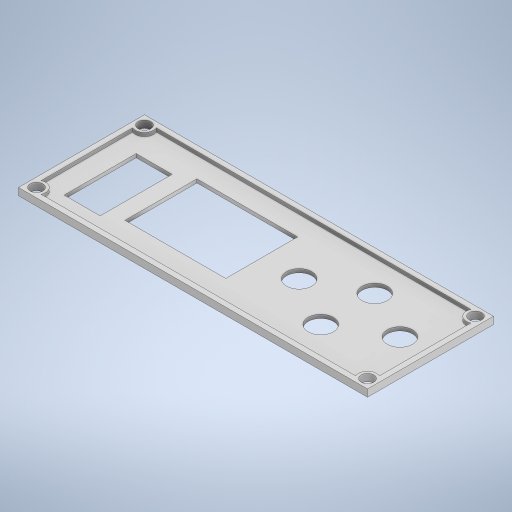
# Autodesk Inventor part: tampa_lcd_botoes
Saved by Autodesk Inventor 2024.3 (Build 283343000, 343)
## iProperties
Created: 2025-02-25
Part Number: tampa_lcd_botoes
Material: Genérico
Document SubType Name: Modeling
Designer: lostv
Density: 1 g/cm^3
Appearance: Padrão
Author: lostv
Autodesk Inventor part; units mm, degrees
ref_plane "YZ Plane" through (0, 0, 0) normal (1, 0, 0) x (0, 1, 0)
ref_plane "XZ Plane" through (0, 0, 0) normal (0, 1, 0) x (-1, 0, 0)
ref_plane "XY Plane" through (0, 0, 0) normal (0, 0, 1) x (1, 0, 0)
sketch "Esboço1" plane through (0, 0, 0) normal (0, 1, 0) x (-1, 0, 0)
  line L0 (-48.4004, 17.271) -> (48.6103, 17.271)
  line L1 (48.6103, 17.271) -> (48.6103, -17.729)
  line L2 (48.6103, -17.729) -> (-48.4004, -17.729)
  line L3 (-48.4004, -17.729) -> (-48.4004, 17.271)
  line L4 (-51.9004, -19.229) -> (-51.9004, 19.271)
  line L5 (-51.9004, 19.271) -> (52.1103, 19.271)
  line L6 (-51.9004, -19.229) -> (52.1103, -19.229)
  line L7 (52.1103, -19.229) -> (52.1103, 19.271)
  circle A0 centre (-45.9004, 14.771) radius 1.75
  circle A1 centre (-45.9004, 14.771) radius 2.5
  circle A2 centre (-45.9004, -15.229) radius 1.75
  circle A3 centre (-45.9004, -15.229) radius 2.5
  circle A4 centre (46.1103, 14.771) radius 2.5
  circle A5 centre (46.1103, 14.771) radius 1.75
  circle A6 centre (46.1103, -15.229) radius 2.5
  circle A7 centre (46.1103, -15.229) radius 1.75
  line L8 (26.9024, 10.578) -> (26.9024, -11.7995)
  line L9 (-30.4004, -2.229) -> (-20.4004, -2.229)
  line L10 (-20.4004, -2.229) -> (-20.4004, -12.229)
  line L11 (-20.4004, -12.229) -> (-30.4004, -12.229)
  line L12 (-30.4004, -12.229) -> (-30.4004, -2.229)
  line L13 (-6.4004, 4.271) -> (-6.4004, -5.729)
  line L14 (-16.4004, 4.271) -> (-6.4004, 4.271)
  line L15 (-16.4004, -5.729) -> (-16.4004, 4.271)
  line L16 (-6.4004, -5.729) -> (-16.4004, -5.729)
  line L17 (-20.4004, 12.271) -> (-20.4004, 2.271)
  line L18 (-30.4004, 12.271) -> (-20.4004, 12.271)
  line L19 (-30.4004, 2.271) -> (-30.4004, 12.271)
  line L20 (-20.4004, 2.271) -> (-30.4004, 2.271)
  line L21 (-34.4004, 4.271) -> (-34.4004, -5.729)
  line L22 (-44.4004, 4.271) -> (-34.4004, 4.271)
  line L23 (-44.4004, -5.729) -> (-44.4004, 4.271)
  line L24 (-34.4004, -5.729) -> (-44.4004, -5.729)
  line L25 (31.4236, 11.771) -> (41.4236, 11.771)
  line L26 (41.4236, 11.771) -> (41.4236, -8.229)
  line L27 (41.4236, -8.229) -> (31.4236, -8.229)
  line L28 (31.4236, -8.229) -> (31.4236, 11.771)
  circle A8 centre (-25.4004, 7.271) radius 3.5
  circle A9 centre (-11.4004, -0.729) radius 3.5
  circle A10 centre (-25.4004, -7.729) radius 3.5
  circle A11 centre (-39.4004, -0.729) radius 3.5
  line L29 (-43.6091, 15.771) -> (43.819, 15.771)
  line L30 (-46.9004, -12.9377) -> (-46.9004, 12.4797)
  line L31 (43.819, -16.229) -> (-43.6091, -16.229)
  line L32 (47.1103, 12.4797) -> (47.1103, -12.9377)
  circle A12 centre (0.1524, 12.1393) radius 1.25
  circle A13 centre (25.6524, -13.3607) radius 1.25
  circle A14 centre (25.6524, 12.1393) radius 1.25
  circle A15 centre (0.1524, -13.3607) radius 1.25
  circle A16 centre (0.1524, -13.3607) radius 2
  circle A17 centre (0.1524, 12.1393) radius 2
  circle A18 centre (25.6524, 12.1393) radius 2
  circle A19 centre (25.6524, -13.3607) radius 2
  line L33 (3.9024, 13.3893) -> (21.9024, 13.3893)
  line L34 (21.9024, 13.3893) -> (21.9024, 6.3893)
  line L35 (21.9024, 6.3893) -> (3.9024, 6.3893)
  line L36 (3.9024, 6.3893) -> (3.9024, 13.3893)
  line L37 (-1.0976, -11.7995) -> (-1.0976, 10.578)
  line L38 (-1.0976, 12.1393) -> (-1.0976, 12.271)
  line L39 (1.7137, 13.3893) -> (24.0912, 13.3893)
  line L40 (26.9024, -14.6107) -> (25.6524, -14.6107)
  line L41 (24.0912, -14.6107) -> (1.7137, -14.6107)
  line L42 (0.1524, -14.6107) -> (-1.0976, -14.6107)
  line L43 (-1.0976, 9.3893) -> (26.9024, 9.3893)
  line L44 (26.9024, 9.3893) -> (26.9024, -10.6107)
  line L45 (26.9024, -10.6107) -> (-1.0976, -10.6107)
  line L46 (-1.0976, -10.6107) -> (-1.0976, 9.3893)
  point P0 (0, 0)
  point P1 (-4.4505, -19.229)
  point P2 (-25.4004, -2.229)
  point P3 (12.9024, 6.3893)
  point P4 (12.9024, 13.3893)
  point P5 (26.9024, -10.6107)
  point P6 (-1.0976, -10.6107)
  dimension "d35" = 2.5
  dimension "d36" = 2.5
  dimension "d38" = 2.5
  dimension "d0" = 3.5
  dimension "d1" = 2
  dimension "d2" = 3.5
  dimension "d3" = 3.5
  dimension "d4" = 5
  dimension "d5" = 3.5
  dimension "d6" = 5
  dimension "d7" = 5
  dimension "d8" = 3.5
  dimension "d9" = 5
  dimension "d10" = 3.5
  dimension "d11" = 104.0106
  dimension "d12" = 38.5
  dimension "d13" = 28
  dimension "d14" = 10
  dimension "d15" = 10
  dimension "d16" = 10
  dimension "d17" = 10
  dimension "d18" = 10
  dimension "d19" = 10
  dimension "d20" = 10
  dimension "d21" = 10
  dimension "d22" = 10
  dimension "d23" = 20
  dimension "d24" = 4
  dimension "d25" = 4
  dimension "d26" = 4
  dimension "d27" = 4
  dimension "d28" = 5.5
  dimension "d29" = 7
  dimension "d30" = 7
  dimension "d31" = 7
  dimension "d32" = 7
  dimension "d33" = 1.5
  dimension "d34" = 4.5
  dimension "d37" = 2.5
  dimension "d39" = 4
  dimension "d40" = 4
  dimension "d41" = 4
  dimension "d42" = 4
  dimension "d43" = 5
  dimension "d44" = 7
  dimension "d47" = 2.3817
  dimension "d48" = 28
  dimension "d49" = 4
  dimension "d50" = 4
  constraints: 94 end point, 23 parallel, 17 centre point, 16 point on circle, 14 horizontal, 10 perpendicular, 8 coincident, 8 tangent, 3 midpoint, 3 vertical, 2 collinear, 2 point on line, 2 vertical alignment, 1 horizontal alignment, 6 other
  measures "d0" distance between parallel lines of L4 L3
  measures "d1" distance between parallel lines of L5 L0
  measures "d2" distance between parallel lines of L7 L1
  measures "d3" diameter of A0
  measures "d4" diameter of A1
  measures "d5" diameter of A2
  measures "d6" diameter of A3
  measures "d7" diameter of A4
  measures "d8" diameter of A5
  measures "d9" diameter of A6
  measures "d10" diameter of A7
  measures "d11" distance between parallel lines of L7 L4
  measures "d12" distance between parallel lines of L6 L5
  measures "d13" distance of L40.start L42.end
  measures "d14" distance of L10.end L11.end
  measures "d15" distance of L10.start L10.end
  measures "d16" distance of L13.end L16.end
  measures "d17" distance of L14.end L13.end
  measures "d18" distance of L17.end L19.start
  measures "d19" distance of L17.start L17.end
  measures "d20" distance of L21.end L24.end
  measures "d21" distance of L21.start L21.end
  measures "d22" distance of L26.end L27.end
  measures "d23" distance between parallel lines of L27 L25
  measures "d24" distance between parallel lines of L21 L19
  measures "d25" distance between parallel lines of L21 L12
  measures "d26" distance between parallel lines of L10 L15
  measures "d27" distance between parallel lines of L17 L15
  measures "d28" distance between parallel lines of L0 L25
  measures "d29" diameter of A8
  measures "d30" diameter of A9
  measures "d31" diameter of A10
  measures "d32" diameter of A11
  measures "d33" distance between parallel lines of L0 L29
  measures "d34" distance from line of point (-25.4, -2.229) L20
  measures "d37" diameter of A14
  measures "d39" diameter of A16
  measures "d40" diameter of A17
  measures "d41" diameter of A18
  measures "d42" diameter of A19
  measures "d43" distance between parallel lines of L8 L34
  measures "d44" distance of point (12.902, 6.389) point (12.902, 13.389)
  measures "d47" distance between parallel lines of L29 L33
  measures "d48" distance between parallel lines of L41 L39
  measures "d49" distance between parallel lines of L39 L43
  measures "d50" distance between parallel lines of L41 L45
extrude "Extrusão1" add sketch "Esboço1" along normal blind 2 contours L0 A1 L3 | L0 A4 L29 A1 | A1 | A1 L30 A3 L3 | L0 L1 A4 | A4 | A3 L2 L3 | A3 | L1 A6 L32 A4 | A3 L31 A6 L2 | A6 | L1 L2 A6
extrude "Extrusão2" add sketch "Esboço1" along normal blind 1 contours L29 A4 L32 A6 L31 A3 L30 A1 | L8 L43 L34 L39 A18 | A18 | L8 A19 L41 A16 L37 L45 | L43 L36 L33 L34 | A19 | L43 L37 A17 L39 L36 | A16 | A17 | L9 L10 L11 L12 | L13 L16 L15 L14 | L17 L20 L19 L18 | L21 L24 L23 L22 | A12 | A13 | A14 | A15
